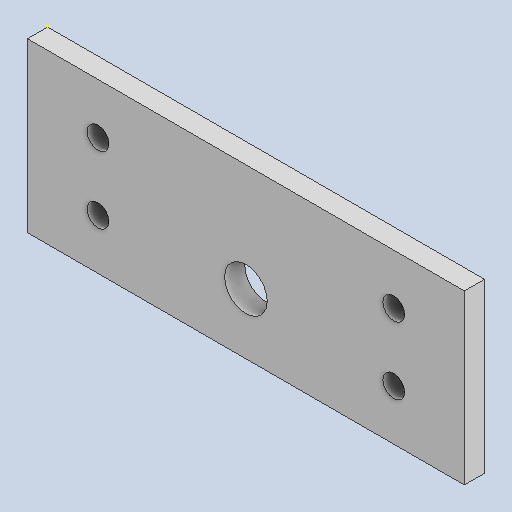
# Autodesk Inventor part: support plate 2
Saved by Autodesk Inventor 2023 (Build 270158000, 158)
## iProperties
Created: 2023-02-07
Part Number: support plate 2
Material: Generic
Document SubType Name: Modeling
Designer: Dell
Density: 1 g/cm^3
Appearance: Default
Author: Dell
Autodesk Inventor part; units mm, degrees
ref_plane "YZ Plane" through (0, 0, 0) normal (1, 0, 0) x (0, 1, 0)
ref_plane "XZ Plane" through (0, 0, 0) normal (0, 1, 0) x (-1, 0, 0)
ref_plane "XY Plane" through (0, 0, 0) normal (0, 0, 1) x (1, 0, 0)
sketch "Sketch1" plane through (0, 0, 0) normal (0, 0, 1) x (1, 0, 0)
  line L0 (0, 0) -> (130, 0)
  line L1 (130, 0) -> (130, 50)
  line L2 (130, 50) -> (0, 50)
  line L3 (0, 50) -> (0, 0)
  line L4 (0, 0) -> (21, 0)
  circle A0 centre (21, 35) radius 3.25
  circle A1 centre (21, 15) radius 3.25
  circle A2 centre (109, 15) radius 3.25
  circle A3 centre (109, 35) radius 3.25
  circle A4 centre (65, 18) radius 6.35
  point P0 (65, 25)
  point P1 (65, 25)
  point P2 (65, 50)
  dimension "d0" = 130
  dimension "d1" = 50
  dimension "d2" = 21
  dimension "d5" = 6.5
  dimension "d6" = 6.5
  dimension "d13" = 20
  dimension "d14" = 15
  dimension "d15" = 21
  dimension "d19" = 360
  dimension "d23" = 65
  dimension "d24" = 12.7
  dimension "d25" = 32
  constraints: 10 end point, 5 centre point, 2 coincident, 2 parallel, 1 horizontal, 1 midpoint, 1 perpendicular, 1 point on line, 9 other
  measures "d0" distance of L2.end L1.end
  measures "d1" distance of L1.end L0.end
  measures "d2" distance of L0.start L4.end
  measures "d5" diameter of A0
  measures "d6" diameter of A1
  measures "d13" distance of A1.centre A0.centre
  measures "d14" distance from line of L2 A0.centre
  measures "d15" distance from line of L3 A0.centre
  measures "d23" distance from line of point (65, 25) L3
  measures "d24" diameter of A4
  measures "d25" distance of point (65, 50) A4.centre
extrude "Extrusion1" add sketch "Sketch1" along normal blind 6 contours L3 L2 L1 L0 | A0 | A2 | A3 | A4
extrude "Extrusion3" cut sketch "Sketch1" along normal blind 10 contours A0 | A2 | A3 | A4
sketch "Sketch4" plane through (0, 50, 0) normal (0, 1, 0) x (1, 0, 0)
  point P0 (0, 0)
body "Solid1"
